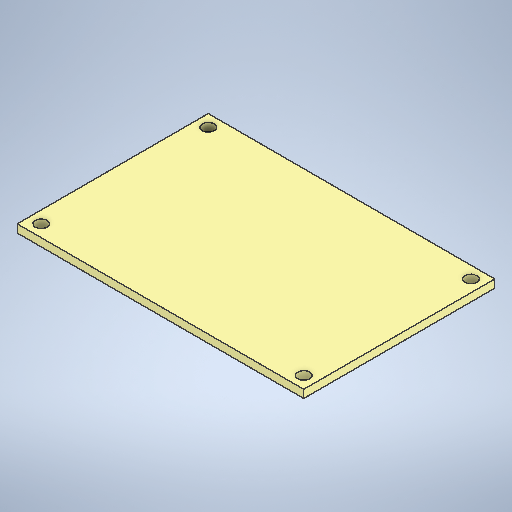
# Autodesk Inventor part: circuitboard
Saved by Autodesk Inventor 2025 (Build 290162000, 162)
## iProperties
Created: 2026-02-25
Part Number: circuitboard
Material: 一般
Document SubType Name: Modeling
Designer: sooo1
Density: 1 g/cm^3
Appearance: 既定
Author: sooo1
Autodesk Inventor part; units mm, degrees
ref_plane "YZ Plane" through (0, 0, 0) normal (1, 0, 0) x (0, 1, 0)
ref_plane "XZ Plane" through (0, 0, 0) normal (0, 1, 0) x (-1, 0, 0)
ref_plane "XY Plane" through (0, 0, 0) normal (0, 0, 1) x (1, 0, 0)
sketch "スケッチ1" plane through (0, 0, 0) normal (0, 1, 0) x (-1, 0, 0)
  line L0 (36, 24) -> (-36, 24)
  line L1 (-36, 24) -> (-36, -24)
  line L2 (-36, -24) -> (36, -24)
  line L3 (36, -24) -> (36, 24)
  line L4 (36, 24) -> (-36, -24) construction
  line L5 (-36, 24) -> (36, -24) construction
  circle A0 centre (33, 21) radius 1.5
  line L6 (50.4, 0) -> (-50.4, 0) construction
  circle A1 centre (33, -21) radius 1.5
  line L7 (0, -33.6) -> (0, 33.6) construction
  circle A2 centre (-33, 21) radius 1.5
  circle A3 centre (-33, -21) radius 1.5
  point P0 (0, 0)
  dimension "d0" = 48
  dimension "d1" = 72
  dimension "d2" = 3
  dimension "d3" = 3
  dimension "d4" = 42
  constraints: 12 end point, 4 centre point, 3 symmetric about line, 2 midpoint, 2 parallel, 1 horizontal, 1 perpendicular, 3 other
  measures "d0" distance of L2.end L0.start
  measures "d1" distance of L1.end L2.end
  measures "d2" diameter of A0
  measures "d3" distance from line of L3 A0.centre
  measures "d4" diameter of A0.centre L6
extrude "押し出し1" add sketch "スケッチ1" along normal blind 2
